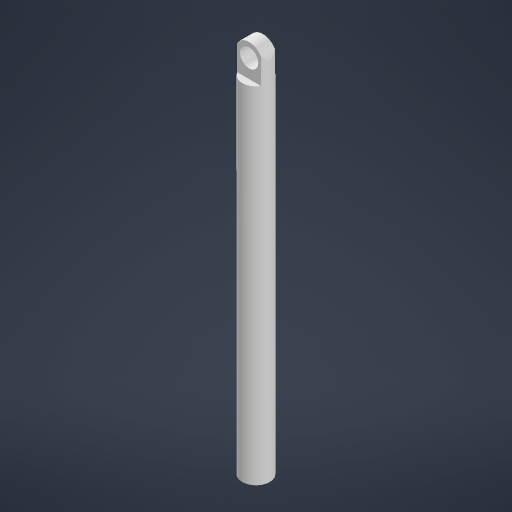
# Autodesk Inventor part: Shaft
Saved by Autodesk Inventor 2023.6 (Build 276521000, 521)
## iProperties
Created: 2026-03-05
Part Number: Shaft
Material: Generic
Document SubType Name: Modeling
Designer: user
Density: 1 g/cm^3
Appearance: Default
Author: user
Autodesk Inventor part; units mm, degrees
ref_plane "YZ Plane" through (0, 0, 0) normal (1, 0, 0) x (0, 1, 0)
ref_plane "XZ Plane" through (0, 0, 0) normal (0, 1, 0) x (-1, 0, 0)
ref_plane "XY Plane" through (0, 0, 0) normal (0, 0, 1) x (1, 0, 0)
sketch "Sketch1" plane through (0, 0, 0) normal (0, 1, 0) x (-1, 0, 0)
  circle A0 centre (0, 0) radius 3
  dimension "d0" = 6
  constraints: 1 centre point, 1 coincident
  measures "d0" diameter of A0
extrude "Extrusion1" add sketch "Sketch1" along normal blind 75
sketch "Sketch2" plane through (0, 75, 0) normal (0, 1, 0) x (1, 0, 0)
  circle A0 centre (0, 0) radius 3 projected
  circle A1 centre (0, 0) radius 3 projected
  line L0 (-2.5981, 1.5) -> (2.5981, 1.5)
  line L1 (2.5981, -1.5) -> (-2.5981, -1.5)
  line L2 (0, -1.5) -> (0, 1.5)
  dimension "d3" = 3
  constraints: 6 end point, 4 point on circle, 2 midpoint, 1 horizontal, 1 parallel
  measures "d3" distance between parallel lines of L1 L0
extrude "Extrusion2" add sketch "Sketch2" along normal blind 7 contours A0 L1 L2 L0 | L0 L2 L1 A0
sketch "Sketch3" plane through (-2.5981, 75, 1.5) normal (0, 0, 1) x (1, 0, 0)
  line L0 (5.5981, -75) -> (5.5981, 7) projected
  line L1 (-0.4019, -75) -> (-0.4019, 7) projected
  line L2 (-0.4019, 4) -> (5.5981, 4)
  circle A0 centre (2.5981, 4) radius 2
  line L3 (0, 7) -> (5.1962, 7) projected
  circle A1 centre (2.5981, 4) radius 3
  line L4 (0, 7) -> (-0.4019, 7) projected
  line L5 (-0.4019, 7) -> (5.5981, 7)
  point P0 (2.5981, -75)
  point P1 (2.5981, 7)
  point P2 (5.5981, 4)
  dimension "d6" = 4
  constraints: 4 end point, 2 centre point, 2 perpendicular, 2 point on line, 2 tangent, 1 coincident, 1 midpoint
  measures "d6" diameter of A0
extrude "Extrusion3" cut sketch "Sketch3" against normal blind 7 contours A1 L3 L5 L0 | A0 L2 | L2 A0 | L1 L4 L3 A1
body "Solid1"
